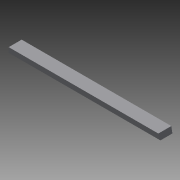
# Autodesk Inventor part: Panel_front
Saved by Autodesk Inventor 2013 (Build 170138000, 138)
## iProperties
Created: 2012-08-20
Part Number: Panel_front
Material: Generic
Document SubType Name: Modeling
Designer: Brandon
Density: 1 g/cm^3
Author: Brandon
Autodesk Inventor part; units mm, degrees
ref_plane "YZ Plane" through (0, 0, 0) normal (1, 0, 0) x (0, 1, 0)
ref_plane "XZ Plane" through (0, 0, 0) normal (0, 1, 0) x (-1, 0, 0)
ref_plane "XY Plane" through (0, 0, 0) normal (0, 0, 1) x (1, 0, 0)
sketch "Sketch1" plane through (0, 0, 0) normal (0, 1, 0) x (-1, 0, 0)
  line L0 (162.815, -12.8435) -> (-162.815, -12.8435)
  line L1 (-162.815, -12.8435) -> (-162.815, 12.8435)
  line L2 (-162.815, 12.8435) -> (162.815, 12.8435)
  line L3 (162.815, 12.8435) -> (162.815, -12.8435)
  point P0 (0, 0)
  point P1 (162.815, 0)
  point P2 (0, -12.8435)
  dimension "d0" = 325.63
  dimension "d2" = 25.687
  constraints: 8 end point, 2 midpoint, 2 parallel, 1 horizontal, 1 horizontal alignment, 1 perpendicular, 1 vertical alignment
  measures "d0" distance of L0.start L0.end
  measures "d2" distance of L2.end L0.start
extrude "Extrusion1" add sketch "Sketch1" along normal blind 12.7
draft "FaceDraft1" angle -10 pull direction (0, -1, 0) faces at (162.815, 8.4667, -4.2812) fixed edges at (162.815, 0, 0)
draft "FaceDraft2" angle -10 pull direction (0, -1, 0) faces at (-162.815, 8.4667, 4.2812) fixed edges at (-162.815, 0, 0)
draft "FaceDraft3" angle 10 pull direction (0, -1, 0) faces at (53.5252, 4.2333, 12.8435) fixed edges at (0, 0, 12.8435)
body "Solid1"
